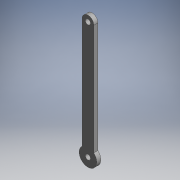
# Autodesk Inventor part: Part3
Saved by Autodesk Inventor 2019.2 (Build 232265000, 265)
## iProperties
Part Number: Part3
Material: Generic
Document SubType Name: Modeling
Designer: richard.girt
Mass: 2.00152 g
Surface Area: 20.3041 cm^2
Volume: 2.00152 cm^3
Density: 1 g/cm^3
Appearance: Default
Author: richard.girt
Autodesk Inventor part; units mm, degrees
ref_plane "YZ Plane" through (0, 0, 0) normal (1, 0, 0) x (0, 1, 0)
ref_plane "XZ Plane" through (0, 0, 0) normal (0, 1, 0) x (-1, 0, 0)
ref_plane "XY Plane" through (0, 0, 0) normal (0, 0, 1) x (1, 0, 0)
sketch "Sketch1" plane through (0, 0, 0) normal (0, 0, 1) x (1, 0, 0)
  circle A0 centre (0, 0) radius 6
  line L0 (0, -2) -> (0, 80) construction
  line L1 (4, -2) -> (4, 80)
  line L2 (-4, 80) -> (-4, -2)
  arc A1 (-4, -2) -> (4, -2) centre (0, -2) ccw
  arc A2 (4, 80) -> (-4, 80) centre (0, 80) ccw
  point P0 (0, 39)
  dimension "d0" = 12
  dimension "d1" = 8
  dimension "d2" = 80
  constraints: 8 end point, 4 point on circle, 4 tangent, 3 centre point, 1 coincident, 1 midpoint, 1 parallel, 1 vertical, 1 vertical alignment
  measures "d0" diameter of A0
  measures "d1" distance between parallel lines of L1 L2
  measures "d2" distance of point (0, 0) L0.end
extrude "Extrusion1" add sketch "Sketch1" along normal mid plane 2.8
sketch "Sketch2" plane through (0, 0, 1.4) normal (0, 0, 1) x (1, 0, 0)
  arc A0 (4, 80) -> (-4, 80) centre (0, 80) ccw construction
  arc A1 (-4, 4.4721) -> (4, 4.4721) centre (0, 0) ccw construction
  circle A2 centre (0, 0) radius 1.75
  circle A3 centre (0, 80) radius 1.75
  line L0 (0, 12.7) -> (0, 5.7) construction
  line L1 (-1.3, 11.4) -> (-1.3, 7)
  line L2 (1.3, 7) -> (1.3, 11.4)
  arc A4 (1.3, 11.4) -> (-1.3, 11.4) centre (0, 11.4) ccw
  arc A5 (-1.3, 7) -> (1.3, 7) centre (0, 7) ccw
  point P0 (0, 9.2)
  dimension "d5" = 7
  dimension "d6" = 2.6
  dimension "d7" = 7
  dimension "d8" = 3.5
  dimension "d9" = 3.5
  constraints: 8 end point, 6 point on circle, 4 centre point, 4 tangent, 2 coincident, 2 point on line, 1 midpoint, 1 parallel, 1 vertical, 1 vertical alignment
  measures "d5" distance of L0.start L0.end
  measures "d6" distance between parallel lines of L1 L2
  measures "d7" distance of A5.centre A2.centre
  measures "d8" diameter of A3
  measures "d9" diameter of A2
extrude "Extrusion2" cut sketch "Sketch2" against normal through all contours A2 | A3
body "Solid1"
